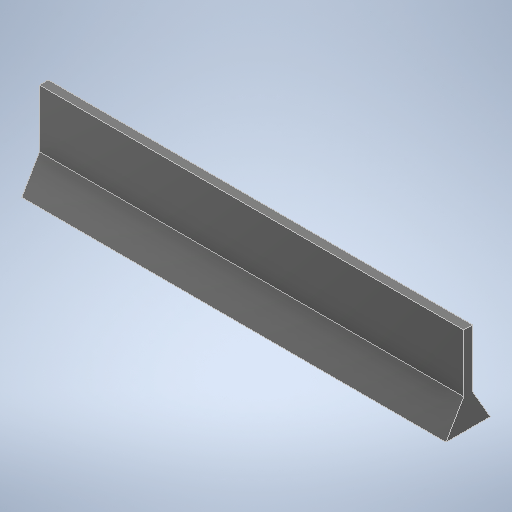
# Autodesk Inventor part: Disk_Barrier
Saved by Autodesk Inventor 2025.1 (Build 291241020, 241B)
## iProperties
Created: 2024-11-16
Part Number: Disk_Barrier
Material: PC/ABS Plastic
Document SubType Name: Modeling
Designer: leon-
Density: 1.1 g/cm^3
Appearance: Smooth - Black
Author: leon-
## iProperties of the stored document Disk_Barrier_3DPrint.ipt
Created: 2024-11-19
Part Number: Disk_Barrier_3DPrint
Material: Generic
Document SubType Name: Modeling
Designer: leon-
Density: 1 g/cm^3
Appearance: Default
Author: leon-
Autodesk Inventor part; units mm, degrees
ref_plane "YZ Plane" through (0, 0, 0) normal (1, 0, 0) x (0, 1, 0)
ref_plane "XZ Plane" through (0, 0, 0) normal (0, 1, 0) x (-1, 0, 0)
ref_plane "XY Plane" through (0, 0, 0) normal (0, 0, 1) x (1, 0, 0)
sketch "Sketch1" plane through (0, 0, 0) normal (0, 0, 1) x (1, 0, 0)
  line L0 (0, 0) -> (240, 0)
  line L1 (240, 0) -> (240, 50)
  line L2 (240, 50) -> (0, 50)
  line L3 (0, 50) -> (0, 0)
  dimension "d0" = 240
  dimension "d1" = 50
  constraints: 8 end point, 2 parallel, 1 horizontal, 1 perpendicular
  measures "d0" distance of L1.end L2.end
  measures "d1" distance of L0.end L1.end
extrude "Extrusion1" add sketch "Sketch1" along normal blind 5
sketch "Sketch2" plane through (0, 0, 0) normal (0, -1, 0) x (1, 0, 0)
  line L0 (0, 0) -> (240, 0) projected
  line L1 (0, 5) -> (240, 5) projected
  line L2 (0, 0) -> (0, 5) projected
  point P0 (48, 2.5)
  point P1 (96, 2.5)
  point P2 (144, 2.5)
  point P3 (192, 2.5)
  point P4 (0, 2.5)
  dimension "d4" = 5
  dimension "d5" = 240
  dimension "d6" = 2.5
  dimension "d7" = 48
  dimension "d8" = 48
  dimension "d9" = 48
  dimension "d10" = 48
  constraints: 3 horizontal alignment, 1 midpoint
  measures "d4" distance between parallel lines of L0 L1
  measures "d5" distance of L1.start L1.end
  measures "d6" distance from line of point (48, 2.5) L1
  measures "d7" distance of point (0, 2.5) point (48, 2.5)
  measures "d8" distance of point (96, 2.5) point (48, 2.5)
  measures "d9" distance of point (144, 2.5) point (96, 2.5)
  measures "d10" distance of point (192, 2.5) point (144, 2.5)
hole "Hole1" at (48, 0, 2.5) at (96, 0, 2.5) at (144, 0, 2.5) at (192, 0, 2.5) direction (0, 1, 0) diameter 4.8 depth 10
sketch "Sketch3" plane through (0, 0, 0) normal (-1, 0, 0) x (0, 0, 1)
  line L0 (4.9, 0) -> (0.1, 0) projected
  line L1 (0.1, 10) -> (4.9, 10) projected
  line L2 (4.9, 0) -> (0.1, 0) projected
  line L3 (0.1, 10) -> (4.9, 10) projected
  line L4 (0, 0) -> (-10, 0)
  line L5 (-10, 0) -> (0, 17.3205)
  line L6 (0, 50) -> (0, 0) projected
  line L7 (5, 50) -> (5, 0) projected
  line L8 (5, 0) -> (15, 0)
  line L9 (15, 0) -> (5, 17.3205)
  point P0 (66.5733, 11.83)
  dimension "d18" = 10
  dimension "d19" = 60
  constraints: 8 end point, 2 equal length, 2 horizontal, 2 point on line, 1 other
  measures "d18" distance of L4.start L4.end
  measures "d19" angle of L4 L5
extrude "Extrusion2" add sketch "Sketch3" against normal up to surface (240 mm away)
equation "\"d6\" = 0.5 * d4"
equation "\"d7\" = 0.2 * d5"
equation "\"d8\" = d7"
equation "\"d9\" = d7"
equation "\"d10\" = d7"
body "Solid1"
